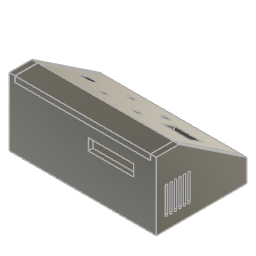
Enclosure_V1 v1 (Autodesk Fusion 360 design; units mm, degrees)
Autodesk Fusion 360 part; units mm, degrees
note: some values were not read from the file. Set by a fixed rule: which sketch regions a step uses; which face or edge a step refers to.
sketch "Sketch1" plane through (0, 0, 0) normal (1, 0, 0) x (0, 1, 0)
  line L0 (0, 0) -> (0, 60)
  line L1 (0, 60) -> (20, 60)
  line L2 (0, 0) -> (80, 0)
  line L3 (80, 0) -> (80, 20)
  line L4 (80, 20) -> (20, 60)
  line L5 (4, 4) -> (4, 55)
  line L6 (76, 17.8593) -> (20.2889, 55)
  line L7 (76, 4) -> (76, 17.8593)
  line L8 (4, 4) -> (76, 4)
  line L9 (0, 55) -> (20, 55)
  line L10 (76, 17.8593) -> (80, 17.8593)
  line L11 (20.2889, 55) -> (20, 55)
  dimension "d1" = 60
  dimension "d2" = 20
  dimension "d3" = 80
  dimension "d4" = 20
  dimension "d6" = 5
  constraint coincident L0.start L2.start
  constraint vertical L0
  constraint perpendicular L0 L1
  constraint perpendicular L0 L2
  constraint perpendicular L2 L3
  constraint coincident L3 L10.end
  constraint perpendicular L3 L10
  constraint coincident L9 L5.end
  constraint parallel L9 L11
  measures "d1" distance of L0.start L0.end
  measures "d2" distance of L0.end L1.end
  measures "d3" distance of L0.start L2.end
  measures "d4" distance of L2.end L3.end
extrude "Extrude1" add sketch "Sketch1" along normal blind 5 makes body 1
extrude "Extrude2" add sketch "Sketch1" against normal blind 60 contours L0 L2 L3 L5 L7 L8 L9 L10 bodies 1
ref_plane "WorkPlane1" through (-60, 40, 30) normal (1, 0, 0) x (0, 0, -1)
mirror "Mirror1" about plane through (-60, 40, 30) normal (1, 0, 0) of bodies 1 merged
extrude "Extrude3" add sketch "Sketch1" against normal blind 119.75 separate body contours L0 L1 L3 L4 L6 L9 L10 L11 makes body 2
sketch "Sketch2" plane through (0, 33.8462, 50.7692) normal (0, 0.5547, 0.83205) x (-1, 0, 0)
  line L0 (0, -55.47) -> (119.75, -55.47)
  line L1 (119.75, -55.47) -> (119.75, 16.641)
  line L2 (119.75, 16.641) -> (0, 16.641)
  circle A0 centre (105.1907, -19.4145) radius 6.25
  line L3 (10, -12.5) -> (35, -12.5)
  line L4 (35, -12.5) -> (35, -27.5)
  line L5 (35, -27.5) -> (10, -27.5)
  line L6 (10, -27.5) -> (10, -12.5)
  line L7 (119.75, -19.4145) -> (0.25, -19.4145) construction
  line L8 (60, -19.4145) -> (60, 0) construction
  line L9 (50, -5) -> (50, -35) construction
  line L10 (50, -35) -> (80, -35) construction
  line L11 (80, -35) -> (80, -5) construction
  circle A1 centre (50, -5) radius 3.75
  circle A2 centre (50, -35) radius 3.75
  circle A3 centre (80, -35) radius 3.75
  circle A4 centre (80, -5) radius 3.75
  line L12 (60, -19.4145) -> (80, -19.4145) construction
  dimension "d17" = 12.5
  dimension "d18" = 15
  dimension "d19" = 25
  dimension "d20" = 7.5
  dimension "d21" = 7.5
  dimension "d22" = 7.5
  dimension "d23" = 7.5
  dimension "d24" = 20
  dimension "d25" = 30
  dimension "d26" = 30
  constraint horizontal L3
  constraint vertical L4
  constraint horizontal L5
  constraint vertical L6
  constraint midpoint L1 L7.start
  constraint perpendicular L6 L7
  constraint coincident A0.centre L7
  constraint midpoint L7 L8.start
  constraint perpendicular L2 L8
  constraint perpendicular L7 L9
  constraint perpendicular L8 L10
  constraint perpendicular L7 L11
  constraint coincident L9.start A1.centre
  constraint coincident L9.end L10.start
  constraint coincident L10.end L11.start
  constraint coincident L11.end A4.centre
  constraint coincident L11 L12.end
  constraint coincident L7 L12.end
  measures "d17" diameter of A0
  measures "d18" distance of L3.start L5.end
  measures "d19" distance of L3.start L3.end
  measures "d20" diameter of A1
  measures "d21" diameter of A2
  measures "d22" diameter of A3
  measures "d23" diameter of A4
  measures "d24" distance of L8.start L12.end
  measures "d25" distance of L9.start L9.end
  measures "d26" distance of L9.end L10.end
extrude "Extrude4" cut sketch "Sketch2" against normal up to surface (4 mm away) bodies 2
move_face "OffsetFaces1" offset -0.125 1 faces at (0, 13.4296, 56.6667) on bodies 2
sketch "Sketch3" plane through (0, 0, 0) normal (0, -1, 0) x (1, 0, 0)
  line L0 (-125, 0) -> (5, 0)
  line L1 (5, 0) -> (5, 60)
  line L2 (5, 60) -> (0, 60)
  line L3 (0, 60) -> (0, 55)
  line L4 (0, 55) -> (-120, 55)
  line L5 (-120, 55) -> (-120, 60)
  line L6 (-120, 60) -> (-125, 60)
  line L7 (-125, 60) -> (-125, 0)
  line L8 (-55, 45) -> (-15, 45)
  line L9 (-15, 45) -> (-15, 35)
  line L10 (-15, 35) -> (-55, 35)
  line L11 (-55, 35) -> (-55, 45)
  constraint horizontal L8
  constraint vertical L9
  constraint horizontal L10
  constraint vertical L11
sketch "Sketch4" plane through (-125, 0, 0) normal (-1, 0, 0) x (0, -1, 0)
  line L0 (-80, 0) -> (0, 0)
  line L1 (0, 0) -> (0, 60)
  line L2 (0, 60) -> (-20, 60)
  line L3 (-20, 60) -> (-80, 20)
  line L4 (-80, 20) -> (-80, 0)
  line L5 (-22.5, 15) -> (-17.5, 15)
  line L6 (-15, 12.5) -> (-15, 7.5)
  line L7 (-17.5, 5) -> (-22.5, 5)
  line L8 (-25, 7.5) -> (-25, 12.5)
  arc A0 (-22.5, 15) -> (-25, 12.5) centre (-22.5, 12.5) ccw
  arc A1 (-15, 12.5) -> (-17.5, 15) centre (-17.5, 12.5) ccw
  arc A2 (-17.5, 5) -> (-15, 7.5) centre (-17.5, 7.5) ccw
  arc A3 (-25, 7.5) -> (-22.5, 5) centre (-22.5, 7.5) ccw
  dimension "d50" = 2.5
  constraint horizontal L5
  constraint vertical L6
  constraint horizontal L7
  constraint vertical L8
  constraint tangent L5 A0
  constraint tangent L8 A0
  constraint tangent L5 A1
  constraint tangent L6 A1
  constraint equal A0 A1
  constraint tangent L6 A2
  constraint tangent L7 A2
  constraint equal A0 A2
  constraint tangent L7 A3
  constraint tangent L8 A3
  constraint equal A0 A3
  measures "d50" radius of A0
sketch "Sketch5" plane through (5, 0, 0) normal (1, 0, 0) x (0, 1, 0)
  line L0 (0, 0) -> (80, 0)
  line L1 (80, 0) -> (80, 20)
  line L2 (80, 20) -> (20, 60)
  line L3 (20, 60) -> (0, 60)
  line L4 (0, 60) -> (0, 0)
  line L5 (10, 11) -> (10, 34)
  line L6 (8, 34) -> (8, 11)
  line L7 (14, 34) -> (14, 11)
  line L8 (12, 11) -> (12, 34)
  line L9 (20, 11) -> (20, 34)
  line L10 (16, 34) -> (16, 11)
  line L11 (18, 11) -> (18, 34)
  line L12 (22, 34) -> (22, 11)
  line L13 (28, 11) -> (28, 34)
  line L14 (26, 11) -> (26, 34)
  line L15 (24, 34) -> (24, 11)
  line L16 (30, 34) -> (30, 11)
  arc A0 (9, 35) -> (8, 34) centre (9, 34) ccw
  arc A1 (13, 35) -> (12, 34) centre (13, 34) ccw
  arc A2 (17, 35) -> (16, 34) centre (17, 34) ccw
  arc A3 (21, 35) -> (20, 34) centre (21, 34) ccw
  arc A4 (25, 35) -> (24, 34) centre (25, 34) ccw
  arc A5 (29, 35) -> (28, 34) centre (29, 34) ccw
  arc A6 (10, 34) -> (9, 35) centre (9, 34) ccw
  arc A7 (14, 34) -> (13, 35) centre (13, 34) ccw
  arc A8 (18, 34) -> (17, 35) centre (17, 34) ccw
  arc A9 (22, 34) -> (21, 35) centre (21, 34) ccw
  arc A10 (26, 34) -> (25, 35) centre (25, 34) ccw
  arc A11 (30, 34) -> (29, 35) centre (29, 34) ccw
  arc A12 (29, 10) -> (30, 11) centre (29, 11) ccw
  arc A13 (28, 11) -> (29, 10) centre (29, 11) ccw
  arc A14 (25, 10) -> (26, 11) centre (25, 11) ccw
  arc A15 (24, 11) -> (25, 10) centre (25, 11) ccw
  arc A16 (21, 10) -> (22, 11) centre (21, 11) ccw
  arc A17 (20, 11) -> (21, 10) centre (21, 11) ccw
  arc A18 (17, 10) -> (18, 11) centre (17, 11) ccw
  arc A19 (16, 11) -> (17, 10) centre (17, 11) ccw
  arc A20 (13, 10) -> (14, 11) centre (13, 11) ccw
  arc A21 (12, 11) -> (13, 10) centre (13, 11) ccw
  arc A22 (9, 10) -> (10, 11) centre (9, 11) ccw
  arc A23 (8, 11) -> (9, 10) centre (9, 11) ccw
  point P0 (8, 10)
  point P1 (10, 10)
  point P2 (16, 10)
  point P3 (18, 10)
  point P4 (24, 10)
  point P5 (26, 10)
  dimension "d30" = 2
  dimension "d31" = 2
  dimension "d32" = 2
  dimension "d33" = 1
  dimension "d34" = 1
  dimension "d35" = 1
  dimension "d36" = 1
  dimension "d37" = 1
  dimension "d38" = 1
  dimension "d39" = 1
  dimension "d40" = 1
  dimension "d41" = 1
  dimension "d42" = 1
  dimension "d43" = 1
  constraint vertical L5
  constraint vertical L6
  constraint vertical L7
  constraint vertical L8
  constraint vertical L11
  constraint vertical L10
  constraint vertical L12
  constraint vertical L9
  constraint vertical L14
  constraint vertical L15
  constraint vertical L16
  constraint vertical L13
  constraint tangent L6 A0
  constraint tangent L8 A1
  constraint tangent L10 A2
  constraint tangent L9 A3
  constraint tangent L15 A4
  constraint tangent L13 A5
  constraint tangent L5 A6
  constraint coincident A0.start A6.end
  constraint tangent L7 A7
  constraint coincident A1.start A7.end
  constraint tangent L11 A8
  constraint coincident A2.start A8.end
  constraint tangent L12 A9
  constraint coincident A3.start A9.end
  constraint tangent L14 A10
  constraint coincident A4.start A10.end
  constraint tangent L16 A11
  constraint equal A10 A11
  constraint coincident A5.start A11.end
  constraint tangent L16 A12
  constraint equal A10 A12
  constraint tangent L13 A13
  constraint equal A10 A13
  constraint coincident A12.start A13.end
  constraint coincident P5 L14
  constraint tangent L14 A14
  constraint equal A10 A14
  constraint coincident P4 L15
  constraint tangent L15 A15
  constraint equal A10 A15
  constraint coincident A14.start A15.end
  constraint tangent L12 A16
  constraint equal A10 A16
  constraint tangent L9 A17
  constraint equal A10 A17
  constraint coincident A16.start A17.end
  constraint coincident P3 L11
  constraint tangent L11 A18
  constraint equal A10 A18
  constraint coincident P2 L10
  constraint tangent L10 A19
  constraint equal A10 A19
  constraint coincident A18.start A19.end
  constraint tangent L7 A20
  constraint equal A10 A20
  constraint tangent L8 A21
  constraint equal A10 A21
  constraint coincident A20.start A21.end
  constraint coincident P1 L5
  constraint tangent L5 A22
  constraint equal A10 A22
  constraint coincident P0 L6
  constraint tangent L6 A23
  constraint equal A10 A23
  constraint coincident A22.start A23.end
  measures "d30" distance of P0 P1
  measures "d31" distance of P2 P3
  measures "d32" distance of P4 P5
  measures "d33" radius of A0
  measures "d34" radius of A1
  measures "d35" radius of A2
  measures "d36" radius of A3
  measures "d37" radius of A4
  measures "d38" radius of A5
  measures "d39" radius of A6
  measures "d40" radius of A7
  measures "d41" radius of A8
  measures "d42" radius of A9
  measures "d43" radius of A10
extrude "Extrude5" cut sketch "Sketch5" against normal up to surface (5 mm away) contours L5 L6 A0 A6 A22 A23 | L7 L8 A1 A7 A20 A21 | L9 L12 A3 A9 A16 A17 | L10 L11 A2 A8 A18 A19 | L13 L16 A5 A11 A12 A13 | L14 L15 A4 A10 A14 A15 bodies 1
extrude "Extrude6" cut sketch "Sketch3" against normal up to surface (4 mm away) contours L8 L9 L10 L11 bodies 1
extrude "Extrude7" cut sketch "Sketch4" against normal up to surface (125 mm away) contours L5 L6 L7 L8 A0 A1 A2 A3 bodies 1
named bodies: "Base", "Lid"
